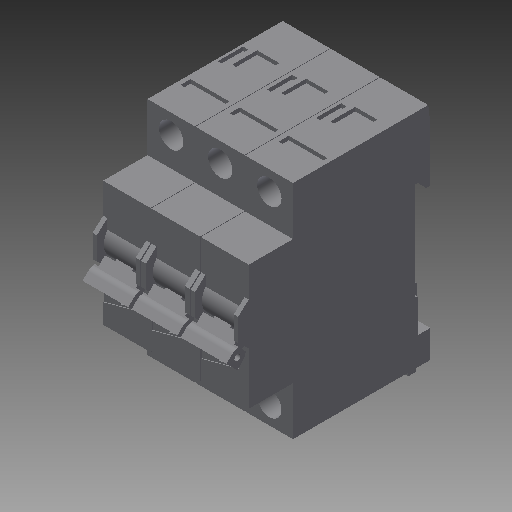
# Autodesk Inventor part: 278851
Saved by Autodesk Inventor 2019.3 (Build 233278000, 278)
## iProperties
Category: PARTsolutions
Company: MOELLER
Created: 2018-10-25
Part Number: 278851
Material: Generic
Catalog Web Link: www.cadenas.de
Description: Miniature Circuit Breakers (MCBs)-
Vendor: MOELLER
Document SubType Name: Modeling
Designer: psadmin
Manufacturer: MOELLER
Mass: 231.527 g
Surface Area: 307.241 cm^2
Volume: 231.527 cm^3
Density: 1 g/cm^3
Appearance: PSOLRGB-175-175-175
PSOL_IDENT_0: {$CADENAS_DATA\23d-libs\moeller\1549\1551\1553\1560.prj},194 {VTYP=3D},{NB=278851},{LINA=278851},{NN=
PSOL_IDENT_1: Miniature Circuit Breakers (MCBs)},{DATE=04.10.2018 12:16:38},{GEOMDATE=04.10.2018 08:29:25},{VERSIO
PSOL_IDENT_2: N=v181004082925},{LINEID=9300},{WBVAR=},{WBNUMERIC=}  {NB=278851},{LINA=278851},{KT=DUMMY},{PFOTO=sg
PSOL_IDENT_3: 53412.jpg},{PLID=278851},{DATA_SHEET=Data sheet},{MANUTYPEDESC=FAZ-B40/3},{DESCSHORT=Miniature circu
PSOL_IDENT_4: it breaker (MCB), 40A, 3p, B-Char, AC},{DESCLONG=Miniature circuit breaker (MCB) FAZ, 3 pole, Trippi
PSOL_IDENT_5: ng characteristic: B, Rated current In: 40 A, Switchgear for industrial and advanced commercial appl
PSOL_IDENT_6: ications},{EAN=4015082788513},{ECLASS_8_1=27-14-19-01},{PACKAGED_WEIGHT=0.350},{DATA_SHEET_=http://d
PSOL_IDENT_7: atasheet.moeller.net/datasheet.php?model=278851&locale=en_GB},{DATA_SHEET_ENG=http://datasheet.moell
PSOL_IDENT_8: er.net/datasheet.php?model=278851&locale=en_GB},{DATA_SHEET_DEU=http://datasheet.moeller.net/datashe
PSOL_IDENT_9: et.php?model=278851&locale=de_DE}
NN: Miniature Circuit Breakers (MCBs)
NB: 278851
NBSYN: $PLID.
LINA: 278851
PFOTO: sg53412.jpg
PLID: 278851
DATA_SHEET: Data sheet
MANUTYPEDESC: FAZ-B40/3
DESCSHORT: Miniature circuit breaker (MCB), 40A, 3p, B-Char, AC
DESCLONG: Miniature circuit breaker (MCB) FAZ, 3 pole, Tripping characteristic: B, Rated current In: 40 A, Switchgear for industrial and advanced commercial applications
EAN: 4015082788513
ECLASS_8_1: 27-14-19-01
PACKAGED_WEIGHT: 0.35
SUPPLIER: MOELLER
ARTICLENO: 278851
BOMINFO: 278851
CREATOR: CADENAS GmbH
Title: 278851
Author: Cadenas PARTsolutions
Autodesk Inventor part; units mm, degrees
ref_plane "YZ Plane" through (0, 0, 0) normal (1, 0, 0) x (0, 1, 0)
ref_plane "XZ Plane" through (0, 0, 0) normal (0, 1, 0) x (-1, 0, 0)
ref_plane "XY Plane" through (0, 0, 0) normal (0, 0, 1) x (1, 0, 0)
sketch "Sketch_1" plane through (26.25, 0, 0) normal (1, 0, 0) x (0, 0, -1)
  line L0 (-63.8, 8.1) -> (-63.8, -0.1)
  line L1 (-63.8, -0.1) -> (-60, -3.6)
  line L2 (-60, -3.6) -> (-60, -22.5)
  line L3 (-60, -22.5) -> (-44, -22.5)
  line L4 (-44, -22.5) -> (-44, -40)
  line L5 (-44, -40) -> (5.5, -40)
  line L6 (5.5, -40) -> (5.5, -30)
  line L7 (5.5, -30) -> (1, -30)
  line L8 (1, -30) -> (1, -18.1)
  arc A0 (1, -18.1) -> (0.7, -17.8) centre (0.7, -18.1) ccw
  line L9 (0.7, -17.8) -> (0, -17.8)
  line L10 (0, -17.8) -> (0, 17.5)
  line L11 (0, 17.5) -> (1, 17.5)
  line L12 (1, 17.5) -> (4, 14.5)
  line L13 (4, 14.5) -> (5.5, 14.5)
  line L14 (5.5, 14.5) -> (5.5, 34)
  line L15 (5.5, 34) -> (4.7633, 40)
  line L16 (4.7633, 40) -> (-44, 40)
  line L17 (-44, 40) -> (-44, 22.5)
  line L18 (-44, 22.5) -> (-60, 22.5)
  line L19 (-60, 22.5) -> (-60, 11.6)
  line L20 (-60, 11.6) -> (-63.8, 8.1)
  constraints: 42 end point, 2 point on circle, 1 centre point
extrude "Extrusion1" add sketch "Sketch_1" along normal mid plane 17.5
sketch "Sketch_22" plane through (26.25, 0, 0) normal (1, 0, 0) x (0, 0, -1)
  line L0 (-59.8, -22.3) -> (-43.8, -22.3)
  line L1 (-43.8, -22.3) -> (-43.8, -39.8)
  line L2 (-43.8, -39.8) -> (5.3, -39.8)
  line L3 (5.3, -39.8) -> (5.3, -30.2)
  line L4 (5.3, -30.2) -> (0.8, -30.2)
  line L5 (0.8, -30.2) -> (0.8, -18.3)
  arc A0 (0.8, -18.3) -> (0.5, -18) centre (0.5, -18.3) ccw
  line L6 (0.5, -18) -> (-0.2, -18)
  line L7 (-0.2, -18) -> (-0.2, 17.7)
  line L8 (-0.2, 17.7) -> (1, 17.7)
  line L9 (1, 17.7) -> (4, 14.7)
  line L10 (4, 14.7) -> (5.3, 14.7)
  line L11 (5.3, 14.7) -> (5.3, 34)
  line L12 (5.3, 34) -> (4.5878, 39.8)
  line L13 (4.5878, 39.8) -> (-43.8, 39.8)
  line L14 (-43.8, 39.8) -> (-43.8, 22.3)
  line L15 (-43.8, 22.3) -> (-59.8, 22.3)
  line L16 (-59.8, 22.3) -> (-59.8, -22.3)
  constraints: 34 end point, 2 point on circle, 1 centre point
extrude "Extrusion2" add sketch "Sketch_22" along normal mid plane 35.4
sketch "Sketch_5" plane through (0, 0, 0) normal (0, 1, 0) x (-1, 0, 0)
  line L0 (-18.55, 19.5) -> (-20.4801, 19.5)
  line L1 (-20.4801, 19.5) -> (-20.4801, 10.4)
  line L2 (-20.4801, 10.4) -> (-18.55, 10.4)
  line L3 (-18.55, 10.4) -> (-18.55, 19.5)
  constraints: 8 end point
extrude "Extrusion3" cut sketch "Sketch_5" along normal mid plane 100
sketch "Sketch_6" plane through (0, 0, 0) normal (0, 1, 0) x (-1, 0, 0)
  line L0 (-22.25, 18) -> (-30.25, 18)
  line L1 (-30.25, 18) -> (-30.25, 9)
  line L2 (-30.25, 9) -> (-22.25, 9)
  line L3 (-22.25, 9) -> (-22.25, 18)
  constraints: 8 end point
extrude "Extrusion4" cut sketch "Sketch_6" along normal mid plane 100
sketch "Sketch_7" plane through (0, 0, 0) normal (0, 1, 0) x (-1, 0, 0)
  line L0 (-19.25, 33.6) -> (-33.25, 33.6)
  line L1 (-33.25, 33.6) -> (-33.25, 30)
  line L2 (-33.25, 30) -> (-19.25, 30)
  line L3 (-19.25, 30) -> (-19.25, 33.6)
  constraints: 8 end point
extrude "Extrusion5" cut sketch "Sketch_7" along normal mid plane 100
sketch "Sketch_8" plane through (0, 0, 0) normal (0, 1, 0) x (-1, 0, 0)
  line L0 (-18.25, 38) -> (-33.75, 38)
  line L1 (-33.75, 38) -> (-33.75, 8)
  line L2 (-33.75, 8) -> (-18.25, 8)
  line L3 (-18.25, 8) -> (-18.25, 38)
  constraints: 8 end point
extrude "Extrusion6" add sketch "Sketch_8" along normal mid plane 77.2
sketch "Sketch_19" plane through (0, 0, 60) normal (0, 0, 1) x (1, 0, 0)
  line L0 (17.55, -15.4982) -> (31.7251, -11.7)
  line L1 (31.7251, -11.7) -> (17.55, -7.9018)
  line L2 (17.55, -7.9018) -> (17.55, -15.4982)
  constraints: 6 end point
extrude "Extrusion7" cut sketch "Sketch_19" along normal mid plane 0.6
sketch "Sketch_20" plane through (0, 0, 60) normal (0, 0, 1) x (1, 0, 0)
  line L0 (23.45, -13.3345) -> (29.55, -11.7)
  line L1 (29.55, -11.7) -> (23.45, -10.0655)
  line L2 (23.45, -10.0655) -> (23.45, -13.3345)
  constraints: 6 end point
extrude "Extrusion8" cut sketch "Sketch_20" against normal blind 0.8
sketch "Sketch_24" plane through (43.95, 0, 0) normal (1, 0, 0) x (0, 0, -1)
  line L0 (-63.8, 8.1) -> (-63.8, -0.1)
  line L1 (-63.8, -0.1) -> (-60, -3.6)
  line L2 (-60, -3.6) -> (-60, -22.5)
  line L3 (-60, -22.5) -> (-44, -22.5)
  line L4 (-44, -22.5) -> (-44, -40)
  line L5 (-44, -40) -> (5.5, -40)
  line L6 (5.5, -40) -> (5.5, -30)
  line L7 (5.5, -30) -> (1, -30)
  line L8 (1, -30) -> (1, -18.1)
  arc A0 (1, -18.1) -> (0.7, -17.8) centre (0.7, -18.1) ccw
  line L9 (0.7, -17.8) -> (0, -17.8)
  line L10 (0, -17.8) -> (0, 17.5)
  line L11 (0, 17.5) -> (1, 17.5)
  line L12 (1, 17.5) -> (4, 14.5)
  line L13 (4, 14.5) -> (5.5, 14.5)
  line L14 (5.5, 14.5) -> (5.5, 34)
  line L15 (5.5, 34) -> (4.7633, 40)
  line L16 (4.7633, 40) -> (-44, 40)
  line L17 (-44, 40) -> (-44, 22.5)
  line L18 (-44, 22.5) -> (-60, 22.5)
  line L19 (-60, 22.5) -> (-60, 11.6)
  line L20 (-60, 11.6) -> (-63.8, 8.1)
  constraints: 42 end point, 2 point on circle, 1 centre point
extrude "Extrusion9" add sketch "Sketch_24" along normal mid plane 17.1
sketch "Sketch_25" plane through (43.95, 0, 0) normal (1, 0, 0) x (0, 0, -1)
  line L0 (1.075, -16.4252) -> (1.075, -44.7)
  line L1 (1.075, -44.7) -> (3.875, -44.7)
  line L2 (3.875, -44.7) -> (3.875, -16.728)
  line L3 (3.875, -16.728) -> (1.575, -15.4001)
  line L4 (1.575, -15.4001) -> (1.075, -16.4252)
  constraints: 10 end point
extrude "Extrusion10" add sketch "Sketch_25" along normal mid plane 11
sketch "Sketch_26" plane through (43.95, 0, 0) normal (1, 0, 0) x (0, 0, -1)
  line L0 (-0.075, -18.9) -> (5.475, -18.9)
  line L1 (5.475, -18.9) -> (5.475, -17.6518)
  line L2 (5.475, -17.6518) -> (1.575, -15.4001)
  line L3 (1.575, -15.4001) -> (0.7215, -17.15)
  line L4 (0.7215, -17.15) -> (-0.075, -17.15)
  line L5 (-0.075, -17.15) -> (-0.075, -18.9)
  constraints: 12 end point
extrude "Extrusion11" add sketch "Sketch_26" along normal mid plane 4
sketch "Sketch_27" plane through (0, 0, 0) normal (0, 0, 1) x (1, 0, 0)
  arc A0 (40.7, -41.95) -> (41.45, -42.7) centre (41.45, -41.95) ccw
  line L0 (41.45, -42.7) -> (46.45, -42.7)
  arc A1 (46.45, -42.7) -> (47.2, -41.95) centre (46.45, -41.95) ccw
  line L1 (47.2, -41.95) -> (47.2, -41.3)
  arc A2 (47.2, -41.3) -> (46.9, -41) centre (46.9, -41.3) ccw
  line L2 (46.9, -41) -> (41, -41)
  arc A3 (41, -41) -> (40.7, -41.3) centre (41, -41.3) ccw
  line L3 (40.7, -41.3) -> (40.7, -41.95)
  constraints: 8 end point, 8 point on circle, 4 centre point
extrude "Extrusion12" cut sketch "Sketch_27" against normal blind 9.156
sketch "Sketch_28" plane through (0, 0, 0) normal (0, 1, 0) x (-1, 0, 0)
  line L0 (-36.25, 19.5) -> (-38.1801, 19.5)
  line L1 (-38.1801, 19.5) -> (-38.1801, 10.4)
  line L2 (-38.1801, 10.4) -> (-36.25, 10.4)
  line L3 (-36.25, 10.4) -> (-36.25, 19.5)
  constraints: 8 end point
extrude "Extrusion13" cut sketch "Sketch_28" along normal mid plane 100
sketch "Sketch_29" plane through (0, 0, 0) normal (0, 1, 0) x (-1, 0, 0)
  line L0 (-39.95, 18) -> (-47.95, 18)
  line L1 (-47.95, 18) -> (-47.95, 9)
  line L2 (-47.95, 9) -> (-39.95, 9)
  line L3 (-39.95, 9) -> (-39.95, 18)
  constraints: 8 end point
extrude "Extrusion14" cut sketch "Sketch_29" along normal mid plane 100
sketch "Sketch_30" plane through (0, 0, 0) normal (0, 1, 0) x (-1, 0, 0)
  line L0 (-36.95, 33.6) -> (-50.95, 33.6)
  line L1 (-50.95, 33.6) -> (-50.95, 30)
  line L2 (-50.95, 30) -> (-36.95, 30)
  line L3 (-36.95, 30) -> (-36.95, 33.6)
  constraints: 8 end point
extrude "Extrusion15" cut sketch "Sketch_30" along normal mid plane 100
sketch "Sketch_31" plane through (0, 0, 0) normal (0, 1, 0) x (-1, 0, 0)
  line L0 (-35.75, 38) -> (-51.25, 38)
  line L1 (-51.25, 38) -> (-51.25, 8)
  line L2 (-51.25, 8) -> (-35.75, 8)
  line L3 (-35.75, 8) -> (-35.75, 38)
  constraints: 8 end point
extrude "Extrusion16" add sketch "Sketch_31" along normal mid plane 77.2
sketch "Sketch_9" plane through (8.55, 0, 0) normal (1, 0, 0) x (0, 0, -1)
  line L0 (-63.8, 8.1) -> (-63.8, -0.1)
  line L1 (-63.8, -0.1) -> (-60, -3.6)
  line L2 (-60, -3.6) -> (-60, -22.5)
  line L3 (-60, -22.5) -> (-44, -22.5)
  line L4 (-44, -22.5) -> (-44, -40)
  line L5 (-44, -40) -> (5.5, -40)
  line L6 (5.5, -40) -> (5.5, -30)
  line L7 (5.5, -30) -> (1, -30)
  line L8 (1, -30) -> (1, -18.1)
  arc A0 (1, -18.1) -> (0.7, -17.8) centre (0.7, -18.1) ccw
  line L9 (0.7, -17.8) -> (0, -17.8)
  line L10 (0, -17.8) -> (0, 17.5)
  line L11 (0, 17.5) -> (1, 17.5)
  line L12 (1, 17.5) -> (4, 14.5)
  line L13 (4, 14.5) -> (5.5, 14.5)
  line L14 (5.5, 14.5) -> (5.5, 34)
  line L15 (5.5, 34) -> (4.7633, 40)
  line L16 (4.7633, 40) -> (-44, 40)
  line L17 (-44, 40) -> (-44, 22.5)
  line L18 (-44, 22.5) -> (-60, 22.5)
  line L19 (-60, 22.5) -> (-60, 11.6)
  line L20 (-60, 11.6) -> (-63.8, 8.1)
  constraints: 42 end point, 2 point on circle, 1 centre point
extrude "Extrusion17" add sketch "Sketch_9" along normal mid plane 17.1
sketch "Sketch_10" plane through (8.55, 0, 0) normal (1, 0, 0) x (0, 0, -1)
  line L0 (1.075, -16.4252) -> (1.075, -44.7)
  line L1 (1.075, -44.7) -> (3.875, -44.7)
  line L2 (3.875, -44.7) -> (3.875, -16.728)
  line L3 (3.875, -16.728) -> (1.575, -15.4001)
  line L4 (1.575, -15.4001) -> (1.075, -16.4252)
  constraints: 10 end point
extrude "Extrusion18" add sketch "Sketch_10" along normal mid plane 11
sketch "Sketch_11" plane through (8.55, 0, 0) normal (1, 0, 0) x (0, 0, -1)
  line L0 (-0.075, -18.9) -> (5.475, -18.9)
  line L1 (5.475, -18.9) -> (5.475, -17.6518)
  line L2 (5.475, -17.6518) -> (1.575, -15.4001)
  line L3 (1.575, -15.4001) -> (0.7215, -17.15)
  line L4 (0.7215, -17.15) -> (-0.075, -17.15)
  line L5 (-0.075, -17.15) -> (-0.075, -18.9)
  constraints: 12 end point
extrude "Extrusion19" add sketch "Sketch_11" along normal mid plane 4
sketch "Sketch_12" plane through (0, 0, 0) normal (0, 0, 1) x (1, 0, 0)
  arc A0 (5.3, -41.95) -> (6.05, -42.7) centre (6.05, -41.95) ccw
  line L0 (6.05, -42.7) -> (11.05, -42.7)
  arc A1 (11.05, -42.7) -> (11.8, -41.95) centre (11.05, -41.95) ccw
  line L1 (11.8, -41.95) -> (11.8, -41.3)
  arc A2 (11.8, -41.3) -> (11.5, -41) centre (11.5, -41.3) ccw
  line L2 (11.5, -41) -> (5.6, -41)
  arc A3 (5.6, -41) -> (5.3, -41.3) centre (5.6, -41.3) ccw
  line L3 (5.3, -41.3) -> (5.3, -41.95)
  constraints: 8 end point, 8 point on circle, 4 centre point
extrude "Extrusion20" cut sketch "Sketch_12" along normal mid plane 10
sketch "Sketch_2" plane through (0, 0, 0) normal (0, 0, 1) x (1, 0, 0)
  line L0 (2.55, -40) -> (2.55, -50)
  line L1 (2.55, -50) -> (49.95, -50)
  line L2 (49.95, -50) -> (49.95, -40)
  line L3 (49.95, -40) -> (48.95, -40)
  line L4 (48.95, -40) -> (48.95, -48)
  line L5 (48.95, -48) -> (38.95, -48)
  line L6 (38.95, -48) -> (38.95, -40)
  line L7 (38.95, -40) -> (37.95, -40)
  line L8 (37.95, -40) -> (37.95, -48)
  line L9 (37.95, -48) -> (14.55, -48)
  line L10 (14.55, -48) -> (14.55, -40)
  line L11 (14.55, -40) -> (13.55, -40)
  line L12 (13.55, -40) -> (13.55, -48)
  line L13 (13.55, -48) -> (3.55, -48)
  line L14 (3.55, -48) -> (3.55, -40)
  line L15 (3.55, -40) -> (2.55, -40)
  constraints: 32 end point
extrude "Extrusion21" cut sketch "Sketch_2" along normal mid plane 10
sketch "Sketch_3" plane through (0, 0, 0) normal (0, 1, 0) x (-1, 0, 0)
  line L0 (-1.55, 33.6) -> (-15.55, 33.6)
  line L1 (-15.55, 33.6) -> (-15.55, 30)
  line L2 (-15.55, 30) -> (-1.55, 30)
  line L3 (-1.55, 30) -> (-1.55, 33.6)
  constraints: 8 end point
extrude "Extrusion22" cut sketch "Sketch_3" along normal mid plane 100
sketch "Sketch_4" plane through (0, 0, 0) normal (0, 1, 0) x (-1, 0, 0)
  line L0 (-4.55, 18) -> (-12.55, 18)
  line L1 (-12.55, 18) -> (-12.55, 9)
  line L2 (-12.55, 9) -> (-4.55, 9)
  line L3 (-4.55, 9) -> (-4.55, 18)
  constraints: 8 end point
extrude "Extrusion23" cut sketch "Sketch_4" along normal mid plane 100
sketch "Sketch_21" plane through (0, 0, 0) normal (0, 1, 0) x (-1, 0, 0)
  line L0 (-0.85, 19.5) -> (-2.7801, 19.5)
  line L1 (-2.7801, 19.5) -> (-2.7801, 10.4)
  line L2 (-2.7801, 10.4) -> (-0.85, 10.4)
  line L3 (-0.85, 10.4) -> (-0.85, 19.5)
  constraints: 8 end point
extrude "Extrusion24" cut sketch "Sketch_21" along normal mid plane 100
sketch "Sketch_32" plane through (0, 0, 0) normal (0, 1, 0) x (-1, 0, 0)
  line L0 (-0.25, 38) -> (-15.75, 38)
  line L1 (-15.75, 38) -> (-15.75, 8)
  line L2 (-15.75, 8) -> (-0.25, 8)
  line L3 (-0.25, 8) -> (-0.25, 38)
  constraints: 8 end point
extrude "Extrusion25" add sketch "Sketch_32" along normal mid plane 77.2
sketch "Sketch_13" plane through (0, 0, 0) normal (0, 1, 0) x (-1, 0, 0)
  line L0 (-1.55, 70) -> (-50.95, 70)
  line L1 (-50.95, 70) -> (-50.95, 60)
  line L2 (-50.95, 60) -> (-36.95, 60)
  line L3 (-36.95, 60) -> (-36.95, 65)
  line L4 (-36.95, 65) -> (-33.25, 65)
  line L5 (-33.25, 65) -> (-33.25, 60)
  line L6 (-33.25, 60) -> (-19.25, 60)
  line L7 (-19.25, 60) -> (-19.25, 65)
  line L8 (-19.25, 65) -> (-15.55, 65)
  line L9 (-15.55, 65) -> (-15.55, 60)
  line L10 (-15.55, 60) -> (-1.55, 60)
  line L11 (-1.55, 60) -> (-1.55, 70)
  constraints: 24 end point
extrude "Extrusion26" cut sketch "Sketch_13" along normal mid plane 40
sketch "Sketch_14" plane through (26.25, 0, 0) normal (1, 0, 0) x (0, 0, -1)
  circle A0 centre (-55, 4) radius 6.35
  constraints: 1 centre point
extrude "Extrusion27" add sketch "Sketch_14" along normal mid plane 14
sketch "Sketch_15" plane through (43.95, 0, 0) normal (1, 0, 0) x (0, 0, -1)
  circle A0 centre (-55, 4) radius 6.35
  constraints: 1 centre point
extrude "Extrusion28" add sketch "Sketch_15" along normal mid plane 14
sketch "Sketch_16" plane through (8.55, 0, 0) normal (1, 0, 0) x (0, 0, -1)
  circle A0 centre (-55, 4) radius 6.35
  constraints: 1 centre point
extrude "Extrusion29" add sketch "Sketch_16" along normal mid plane 14
sketch "Sketch_17" plane through (26.25, 0, 0) normal (1, 0, 0) x (0, 0, -1)
  line L0 (-63.6974, -1.869) -> (-60.8581, -4.7082)
  line L1 (-60.8581, -4.7082) -> (-57.6762, -1.5262)
  line L2 (-57.6762, -1.5262) -> (-60.5154, 1.313)
  line L3 (-60.5154, 1.313) -> (-63.6974, -1.869)
  constraints: 8 end point
extrude "Extrusion30" add sketch "Sketch_17" along normal mid plane 6
sketch "Sketch_18" plane through (26.25, 0, 0) normal (1, 0, 0) x (0, 0, -1)
  line L0 (-63.6974, -1.869) -> (-60.8581, -4.7082)
  line L1 (-60.8581, -4.7082) -> (-58.3126, -2.1626)
  line L2 (-58.3126, -2.1626) -> (-61.1518, 0.6766)
  line L3 (-61.1518, 0.6766) -> (-63.6974, -1.869)
  constraints: 8 end point
extrude "Extrusion31" add sketch "Sketch_18" along normal mid plane 13.5
sketch "Sketch_33" plane through (26.25, 0, 0) normal (1, 0, 0) x (0, 0, -1)
  line L0 (-67.7279, -4.7681) -> (-63.7681, -8.7279)
  line L1 (-63.7681, -8.7279) -> (-61.7882, -6.748)
  arc A0 (-61.7882, -6.748) -> (-60.9686, -4.8186) centre (-63.7681, -4.7681) ccw
  line L2 (-60.9686, -4.8186) -> (-60.6039, -4.454)
  line L3 (-60.6039, -4.454) -> (-63.4431, -1.6147)
  line L4 (-63.4431, -1.6147) -> (-63.7966, -1.9682)
  arc A1 (-63.7966, -1.9682) -> (-65.748, -2.7882) centre (-63.7681, -4.7681) ccw
  line L5 (-65.748, -2.7882) -> (-67.7279, -4.7681)
  constraints: 12 end point, 4 point on circle, 2 centre point
extrude "Extrusion32" add sketch "Sketch_33" along normal mid plane 16.5
sketch "Sketch_34" plane through (0, 0, 60) normal (0, 0, 1) x (1, 0, 0)
  line L0 (-0.2, -15.4982) -> (13.9751, -11.7)
  line L1 (13.9751, -11.7) -> (-0.2, -7.9018)
  line L2 (-0.2, -7.9018) -> (-0.2, -15.4982)
  constraints: 6 end point
extrude "Extrusion33" cut sketch "Sketch_34" along normal mid plane 0.6
sketch "Sketch_35" plane through (0, 0, 60) normal (0, 0, 1) x (1, 0, 0)
  line L0 (5.75, -13.3345) -> (11.85, -11.7)
  line L1 (11.85, -11.7) -> (5.75, -10.0655)
  line L2 (5.75, -10.0655) -> (5.75, -13.3345)
  constraints: 6 end point
extrude "Extrusion34" cut sketch "Sketch_35" against normal blind 0.8
sketch "Sketch_36" plane through (0, 0, 60) normal (0, 0, 1) x (1, 0, 0)
  line L0 (35.2, -15.4982) -> (49.3751, -11.7)
  line L1 (49.3751, -11.7) -> (35.2, -7.9018)
  line L2 (35.2, -7.9018) -> (35.2, -15.4982)
  constraints: 6 end point
extrude "Extrusion35" cut sketch "Sketch_36" along normal mid plane 0.6
sketch "Sketch_37" plane through (0, 0, 60) normal (0, 0, 1) x (1, 0, 0)
  line L0 (41.15, -13.3345) -> (47.25, -11.7)
  line L1 (47.25, -11.7) -> (41.15, -10.0655)
  line L2 (41.15, -10.0655) -> (41.15, -13.3345)
  constraints: 6 end point
extrude "Extrusion36" cut sketch "Sketch_37" against normal blind 0.8
sketch "Sketch_38" plane through (8.55, 0, 0) normal (1, 0, 0) x (0, 0, -1)
  line L0 (-63.6974, -1.869) -> (-60.8581, -4.7082)
  line L1 (-60.8581, -4.7082) -> (-57.6762, -1.5262)
  line L2 (-57.6762, -1.5262) -> (-60.5154, 1.313)
  line L3 (-60.5154, 1.313) -> (-63.6974, -1.869)
  constraints: 8 end point
extrude "Extrusion37" add sketch "Sketch_38" along normal mid plane 6
sketch "Sketch_39" plane through (43.95, 0, 0) normal (1, 0, 0) x (0, 0, -1)
  line L0 (-63.6974, -1.869) -> (-60.8581, -4.7082)
  line L1 (-60.8581, -4.7082) -> (-57.6762, -1.5262)
  line L2 (-57.6762, -1.5262) -> (-60.5154, 1.313)
  line L3 (-60.5154, 1.313) -> (-63.6974, -1.869)
  constraints: 8 end point
extrude "Extrusion38" add sketch "Sketch_39" along normal mid plane 6
sketch "Sketch_40" plane through (8.55, 0, 0) normal (1, 0, 0) x (0, 0, -1)
  line L0 (-63.6974, -1.869) -> (-60.8581, -4.7082)
  line L1 (-60.8581, -4.7082) -> (-58.3126, -2.1626)
  line L2 (-58.3126, -2.1626) -> (-61.1518, 0.6766)
  line L3 (-61.1518, 0.6766) -> (-63.6974, -1.869)
  constraints: 8 end point
extrude "Extrusion39" add sketch "Sketch_40" along normal mid plane 13.5
sketch "Sketch_41" plane through (43.95, 0, 0) normal (1, 0, 0) x (0, 0, -1)
  line L0 (-63.6974, -1.869) -> (-60.8581, -4.7082)
  line L1 (-60.8581, -4.7082) -> (-58.3126, -2.1626)
  line L2 (-58.3126, -2.1626) -> (-61.1518, 0.6766)
  line L3 (-61.1518, 0.6766) -> (-63.6974, -1.869)
  constraints: 8 end point
extrude "Extrusion40" add sketch "Sketch_41" along normal mid plane 13.5
sketch "Sketch_42" plane through (8.55, 0, 0) normal (1, 0, 0) x (0, 0, -1)
  line L0 (-67.7279, -4.7681) -> (-63.7681, -8.7279)
  line L1 (-63.7681, -8.7279) -> (-61.7882, -6.748)
  arc A0 (-61.7882, -6.748) -> (-60.9686, -4.8186) centre (-63.7681, -4.7681) ccw
  line L2 (-60.9686, -4.8186) -> (-60.6039, -4.454)
  line L3 (-60.6039, -4.454) -> (-63.4431, -1.6147)
  line L4 (-63.4431, -1.6147) -> (-63.7966, -1.9682)
  arc A1 (-63.7966, -1.9682) -> (-65.748, -2.7882) centre (-63.7681, -4.7681) ccw
  line L5 (-65.748, -2.7882) -> (-67.7279, -4.7681)
  constraints: 12 end point, 4 point on circle, 2 centre point
extrude "Extrusion41" add sketch "Sketch_42" along normal mid plane 16.5
sketch "Sketch_43" plane through (43.95, 0, 0) normal (1, 0, 0) x (0, 0, -1)
  line L0 (-67.7279, -4.7681) -> (-63.7681, -8.7279)
  line L1 (-63.7681, -8.7279) -> (-61.7882, -6.748)
  arc A0 (-61.7882, -6.748) -> (-60.9686, -4.8186) centre (-63.7681, -4.7681) ccw
  line L2 (-60.9686, -4.8186) -> (-60.6039, -4.454)
  line L3 (-60.6039, -4.454) -> (-63.4431, -1.6147)
  line L4 (-63.4431, -1.6147) -> (-63.7966, -1.9682)
  arc A1 (-63.7966, -1.9682) -> (-65.748, -2.7882) centre (-63.7681, -4.7681) ccw
  line L5 (-65.748, -2.7882) -> (-67.7279, -4.7681)
  constraints: 12 end point, 4 point on circle, 2 centre point
extrude "Extrusion42" add sketch "Sketch_43" along normal mid plane 16.5
sketch "Sketch_44" plane through (26.25, 0, 0) normal (1, 0, 0) x (0, 0, -1)
  circle A0 centre (-63.7681, -4.7681) radius 1.11
  constraints: 1 centre point
extrude "Extrusion43" cut sketch "Sketch_44" along normal mid plane 100
sketch "Sketch44" plane through (0, 22.5, 44) normal (0, 0, 1) x (1, 0, 0)
  point P0 (8.55, 10.5)
hole "Hole1" at (8.55, 33, 44) direction (0, 0, -1) diameter 8.8 depth 9
sketch "Sketch45" plane through (17.5, 22.5, 44) normal (0, 0, 1) x (1, 0, 0)
  point P0 (8.75, 10.5)
hole "Hole2" at (26.25, 33, 44) direction (0, 0, -1) diameter 8.8 depth 9
sketch "Sketch46" plane through (35.4, 22.5, 44) normal (0, 0, 1) x (1, 0, 0)
  point P0 (8.55, 10.5)
hole "Hole3" at (43.95, 33, 44) direction (0, 0, -1) diameter 8.8 depth 9
sketch "Sketch47" plane through (0, -40, 44) normal (0, 0, 1) x (1, 0, 0)
  point P0 (8.55, 7)
hole "Hole4" at (8.55, -33, 44) direction (0, 0, -1) diameter 8.8 depth 9
sketch "Sketch48" plane through (17.5, -40, 44) normal (0, 0, 1) x (1, 0, 0)
  point P0 (8.75, 7)
hole "Hole5" at (26.25, -33, 44) direction (0, 0, -1) diameter 8.8 depth 9
sketch "Sketch49" plane through (35.4, -40, 44) normal (0, 0, 1) x (1, 0, 0)
  point P0 (8.55, 7)
hole "Hole6" at (43.95, -33, 44) direction (0, 0, -1) diameter 8.8 depth 9
sketch "Sketch_47" plane through (0, 0, 44) normal (0, 0, 1) x (1, 0, 0)
  line L0 (5.2414, 35.2479) -> (7.4893, 33)
  line L1 (7.4893, 33) -> (6.3333, 31.844)
  arc A0 (6.3333, 31.844) -> (7.394, 30.7833) centre (8.55, 33) ccw
  line L2 (7.394, 30.7833) -> (8.55, 31.9393)
  line L3 (8.55, 31.9393) -> (10.7979, 29.6914)
  arc A1 (10.7979, 29.6914) -> (11.8586, 30.7521) centre (8.55, 33) ccw
  line L4 (11.8586, 30.7521) -> (9.6107, 33)
  line L5 (9.6107, 33) -> (10.7667, 34.156)
  arc A2 (10.7667, 34.156) -> (9.706, 35.2167) centre (8.55, 33) ccw
  line L6 (9.706, 35.2167) -> (8.55, 34.0607)
  line L7 (8.55, 34.0607) -> (6.3021, 36.3086)
  arc A3 (6.3021, 36.3086) -> (5.2414, 35.2479) centre (8.55, 33) ccw
  constraints: 16 end point, 8 point on circle, 4 centre point
extrude "Extrusion44" cut sketch "Sketch_47" against normal blind 10.6
sketch "Sketch_48" plane through (0, 0, 44) normal (0, 0, 1) x (1, 0, 0)
  line L0 (5.2414, -30.7521) -> (7.4893, -33)
  line L1 (7.4893, -33) -> (6.3333, -34.156)
  arc A0 (6.3333, -34.156) -> (7.394, -35.2167) centre (8.55, -33) ccw
  line L2 (7.394, -35.2167) -> (8.55, -34.0607)
  line L3 (8.55, -34.0607) -> (10.7979, -36.3086)
  arc A1 (10.7979, -36.3086) -> (11.8586, -35.2479) centre (8.55, -33) ccw
  line L4 (11.8586, -35.2479) -> (9.6107, -33)
  line L5 (9.6107, -33) -> (10.7667, -31.844)
  arc A2 (10.7667, -31.844) -> (9.706, -30.7833) centre (8.55, -33) ccw
  line L6 (9.706, -30.7833) -> (8.55, -31.9393)
  line L7 (8.55, -31.9393) -> (6.3021, -29.6914)
  arc A3 (6.3021, -29.6914) -> (5.2414, -30.7521) centre (8.55, -33) ccw
  constraints: 16 end point, 8 point on circle, 4 centre point
extrude "Extrusion45" cut sketch "Sketch_48" against normal blind 10.6
sketch "Sketch_54" plane through (0, 0, 44) normal (0, 0, 1) x (1, 0, 0)
  line L0 (22.9414, 35.2479) -> (25.1893, 33)
  line L1 (25.1893, 33) -> (24.0333, 31.844)
  arc A0 (24.0333, 31.844) -> (25.094, 30.7833) centre (26.25, 33) ccw
  line L2 (25.094, 30.7833) -> (26.25, 31.9393)
  line L3 (26.25, 31.9393) -> (28.4979, 29.6914)
  arc A1 (28.4979, 29.6914) -> (29.5586, 30.7521) centre (26.25, 33) ccw
  line L4 (29.5586, 30.7521) -> (27.3107, 33)
  line L5 (27.3107, 33) -> (28.4667, 34.156)
  arc A2 (28.4667, 34.156) -> (27.406, 35.2167) centre (26.25, 33) ccw
  line L6 (27.406, 35.2167) -> (26.25, 34.0607)
  line L7 (26.25, 34.0607) -> (24.0021, 36.3086)
  arc A3 (24.0021, 36.3086) -> (22.9414, 35.2479) centre (26.25, 33) ccw
  constraints: 16 end point, 8 point on circle, 4 centre point
extrude "Extrusion46" cut sketch "Sketch_54" against normal blind 10.6
sketch "Sketch_55" plane through (0, 0, 44) normal (0, 0, 1) x (1, 0, 0)
  line L0 (22.9414, -30.7521) -> (25.1893, -33)
  line L1 (25.1893, -33) -> (24.0333, -34.156)
  arc A0 (24.0333, -34.156) -> (25.094, -35.2167) centre (26.25, -33) ccw
  line L2 (25.094, -35.2167) -> (26.25, -34.0607)
  line L3 (26.25, -34.0607) -> (28.4979, -36.3086)
  arc A1 (28.4979, -36.3086) -> (29.5586, -35.2479) centre (26.25, -33) ccw
  line L4 (29.5586, -35.2479) -> (27.3107, -33)
  line L5 (27.3107, -33) -> (28.4667, -31.844)
  arc A2 (28.4667, -31.844) -> (27.406, -30.7833) centre (26.25, -33) ccw
  line L6 (27.406, -30.7833) -> (26.25, -31.9393)
  line L7 (26.25, -31.9393) -> (24.0021, -29.6914)
  arc A3 (24.0021, -29.6914) -> (22.9414, -30.7521) centre (26.25, -33) ccw
  constraints: 16 end point, 8 point on circle, 4 centre point
extrude "Extrusion47" cut sketch "Sketch_55" against normal blind 10.6
sketch "Sketch_56" plane through (0, 0, 44) normal (0, 0, 1) x (1, 0, 0)
  line L0 (40.6414, 35.2479) -> (42.8893, 33)
  line L1 (42.8893, 33) -> (41.7333, 31.844)
  arc A0 (41.7333, 31.844) -> (42.794, 30.7833) centre (43.95, 33) ccw
  line L2 (42.794, 30.7833) -> (43.95, 31.9393)
  line L3 (43.95, 31.9393) -> (46.1979, 29.6914)
  arc A1 (46.1979, 29.6914) -> (47.2586, 30.7521) centre (43.95, 33) ccw
  line L4 (47.2586, 30.7521) -> (45.0107, 33)
  line L5 (45.0107, 33) -> (46.1667, 34.156)
  arc A2 (46.1667, 34.156) -> (45.106, 35.2167) centre (43.95, 33) ccw
  line L6 (45.106, 35.2167) -> (43.95, 34.0607)
  line L7 (43.95, 34.0607) -> (41.7021, 36.3086)
  arc A3 (41.7021, 36.3086) -> (40.6414, 35.2479) centre (43.95, 33) ccw
  constraints: 16 end point, 8 point on circle, 4 centre point
extrude "Extrusion48" cut sketch "Sketch_56" against normal blind 10.6
sketch "Sketch_57" plane through (0, 0, 44) normal (0, 0, 1) x (1, 0, 0)
  line L0 (40.6414, -30.7521) -> (42.8893, -33)
  line L1 (42.8893, -33) -> (41.7333, -34.156)
  arc A0 (41.7333, -34.156) -> (42.794, -35.2167) centre (43.95, -33) ccw
  line L2 (42.794, -35.2167) -> (43.95, -34.0607)
  line L3 (43.95, -34.0607) -> (46.1979, -36.3086)
  arc A1 (46.1979, -36.3086) -> (47.2586, -35.2479) centre (43.95, -33) ccw
  line L4 (47.2586, -35.2479) -> (45.0107, -33)
  line L5 (45.0107, -33) -> (46.1667, -31.844)
  arc A2 (46.1667, -31.844) -> (45.106, -30.7833) centre (43.95, -33) ccw
  line L6 (45.106, -30.7833) -> (43.95, -31.9393)
  line L7 (43.95, -31.9393) -> (41.7021, -29.6914)
  arc A3 (41.7021, -29.6914) -> (40.6414, -30.7521) centre (43.95, -33) ccw
  constraints: 16 end point, 8 point on circle, 4 centre point
extrude "Extrusion49" cut sketch "Sketch_57" against normal blind 10.6
sketch "Sketch_23" plane through (26.25, 0, 0) normal (1, 0, 0) x (0, 0, -1)
  circle A0 centre (-63.7681, -4.7681) radius 1.11
  constraints: 1 centre point
extrude "Extrusion50" add sketch "Sketch_23" along normal mid plane 42.9
sketch "Sketch_49" plane through (0, 0, 0) normal (0, 1, 0) x (-1, 0, 0)
  line L0 (-20.8, -1.075) -> (-32, -1.075)
  line L1 (-32, -1.075) -> (-32, -3.875)
  line L2 (-32, -3.875) -> (-20.8, -3.875)
  line L3 (-20.8, -3.875) -> (-20.8, -1.075)
  constraints: 8 end point
extrude "Extrusion51" cut sketch "Sketch_49" against normal blind 50
body "Solid1"
